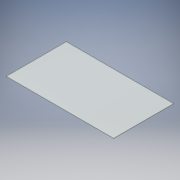
# Autodesk Inventor part: Display Glass
Saved by Autodesk Inventor 2017 SP1 (Build 210196100, 196)
## iProperties
Part Number: Display Glass
Material: Glas
Document SubType Name: Modeling
Designer: u26048
Density: 2.18 g/cm^3
Appearance: Klar
Author: u26048
Autodesk Inventor part; units mm, degrees
ref_plane "YZ Plane" through (0, 0, 0) normal (1, 0, 0) x (0, 1, 0)
ref_plane "XZ Plane" through (0, 0, 0) normal (0, 1, 0) x (-1, 0, 0)
ref_plane "XY Plane" through (0, 0, 0) normal (0, 0, 1) x (1, 0, 0)
sketch "Skizze1" plane through (0, 0, 0) normal (0, 0, 1) x (1, 0, 0)
  line L0 (-77.44, 43.36) -> (77.44, 43.36)
  line L1 (77.44, 43.36) -> (77.44, -43.36)
  line L2 (77.44, -43.36) -> (-77.44, -43.36)
  line L3 (-77.44, -43.36) -> (-77.44, 43.36)
  line L4 (-77.44, 43.36) -> (77.44, 43.36)
  line L5 (77.44, 43.36) -> (77.44, -43.36)
  line L6 (77.44, -43.36) -> (-77.44, -43.36)
  line L7 (-77.44, -43.36) -> (-77.44, 43.36)
  line L8 (-77.44, 43.36) -> (77.44, 43.36)
  line L9 (77.44, 43.36) -> (77.44, -43.36)
  line L10 (77.44, -43.36) -> (-77.44, -43.36)
  line L11 (-77.44, -43.36) -> (-77.44, 43.36)
  point P0 (0, 0)
  point P1 (0, 0)
  point P2 (77.44, 0)
  point P3 (0, 43.36)
  point P4 (0, 0)
  point P5 (77.44, 0)
  point P6 (0, 43.36)
  point P7 (0, 0)
  point P8 (77.44, 0)
  point P9 (0, 43.36)
  dimension "d0" = 154.88
  dimension "d1" = 86.72
  dimension "d2" = 154.88
  dimension "d3" = 86.72
  dimension "d4" = 154.88
  dimension "d5" = 86.72
  constraints: 24 end point, 6 midpoint, 6 parallel, 3 horizontal, 3 horizontal alignment, 3 perpendicular, 3 vertical alignment
  measures "d0" distance between parallel lines of L1 L3
  measures "d1" distance between parallel lines of L2 L0
  measures "d2" distance between parallel lines of L5 L7
  measures "d3" distance between parallel lines of L6 L4
  measures "d4" distance between parallel lines of L9 L11
  measures "d5" distance between parallel lines of L10 L8
extrude "Extrusion1" add sketch "Skizze1" against normal blind 0.7
